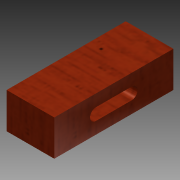
# Autodesk Inventor part: tensioner_wood_block(twb)
Saved by Autodesk Inventor 2015 SP1 (Build 190203100, 203)
## iProperties
Created: 2015-10-09
Part Number: tensioner_wood_block(twb)
Material: Wood (Oak)
Document SubType Name: Modeling
Designer: elilitwack
Density: 0.76 g/cm^3
Appearance: White Oak - Natural Medium Gloss
Mass: 20.4051 g
Surface Area: 77.8206 cm^2
Volume: 26.8488 cm^3
Author: elilitwack
Autodesk Inventor part; units mm, degrees
ref_plane "YZ Plane" through (0, 0, 0) normal (1, 0, 0) x (0, 1, 0)
ref_plane "XZ Plane" through (0, 0, 0) normal (0, 1, 0) x (-1, 0, 0)
ref_plane "XY Plane" through (0, 0, 0) normal (0, 0, 1) x (1, 0, 0)
sketch "tensioner_wood_block_base_sketch" plane through (0, 0, 0) normal (0, 1, 0) x (-1, 0, 0)
  line L0 (0, 0) -> (25.4, 0)
  line L1 (25.4, 0) -> (25.4, -63.5)
  line L2 (25.4, -63.5) -> (0, -63.5)
  line L3 (0, -63.5) -> (0, 0)
  dimension "d0" = 25.4
  dimension "d1" = 63.5
  constraints: 8 end point, 2 parallel, 1 horizontal, 1 perpendicular
  measures "d0" distance of L1.end L2.end
  measures "d1" distance of L0.end L1.end
extrude "base_extrusion" add sketch "tensioner_wood_block_base_sketch" along normal blind 19.05
sketch "tensioner_sketch" plane through (-25.4, 0, -63.5) normal (-1, 0, 0) x (0, 0, 1)
  line L0 (41.275, 9.525) -> (22.225, 9.525) construction
  line L1 (41.275, 12.7) -> (22.225, 12.7)
  line L2 (22.225, 6.35) -> (41.275, 6.35)
  arc A0 (41.275, 6.35) -> (41.275, 12.7) centre (41.275, 9.525) ccw
  arc A1 (22.225, 12.7) -> (22.225, 6.35) centre (22.225, 9.525) ccw
  line L3 (63.5, 0) -> (63.5, 19.05) projected
  line L4 (63.5, 0) -> (0, 0) projected
  line L5 (31.75, 0) -> (31.75, 9.525) construction
  line L6 (31.75, 9.525) -> (31.75, 19.05) construction
  line L7 (0, 19.05) -> (63.5, 19.05) projected
  dimension "d4" = 22.225
  dimension "d5" = 19.05
  dimension "d6" = 6.35
  constraints: 12 end point, 4 point on circle, 4 tangent, 3 midpoint, 2 centre point, 1 collinear, 1 horizontal, 1 parallel
  measures "d4" distance from line of L3 L0.start
  measures "d5" distance of L0.start L0.end
  measures "d6" distance between parallel lines of L1 L2
extrude "tensioner" cut sketch "tensioner_sketch" against normal up to next
equation "\"d0\" = twb_width"
equation "\"d1\" = twb_height"
equation "\"d2\" = twb_length"
equation "\"d4\" = twb_tensioner_from_edge"
equation "\"d5\" = bp_tensioner_height"
equation "\"d6\" = bp_tensioner_width"
equation "\"d7\" = twb_length"
equation "\"bp_thickness\" = 3.048"
equation "\"bp_height\" = gb_mh_seperation + st_outer_diameter"
equation "\"bp_width\" = 6 * st_rivet_distance"
equation "\"bp_axle_height\" = magic_axle_offset + gb_axle_from_edge + gb_to_bottom_of_side_assembly"
equation "\"magic_axle_offset\" = 3.175"
equation "\"bp_tensioner_width\" = 6.35"
equation "\"bp_tensioner_height\" = 19.05"
equation "\"bp_tensioner_from_bottom\" = 50.8"
equation "\"bp_tensioner_from_side\" = 25.4"
equation "\"bp_tensioner_wood_mount_from_tensioner_top\" = 12.7"
equation "\"bp_tensioner_wood_mount_diameter\" = 6.35"
equation "\"gb_mh_seperation\" = 111.1504"
equation "\"gb_mh_diameter\" = 6.35"
equation "\"gb_axle_from_edge\" = 38.1"
equation "\"gb_width\" = 127"
equation "\"gb_bearing_diameter\" = 28.575"
equation "\"gb_to_bottom_of_side_assembly\" = 4.7752"
equation "\"rv_hole_diameter\" = 3.57187"
equation "\"st_outer_diameter\" = 25.4"
equation "\"st_wall_thickness\" = 6.35"
equation "\"st_length\" = 939.8"
equation "\"st_gbmh_from_center\" = 0.5 * gb_mh_seperation"
equation "\"st_cutout_depth_right\" = 342.9"
equation "\"st_cutout_depth_left\" = 342.9"
equation "\"st_rivet_distance\" = 19.05"
equation "\"so_inner_diameter\" = 6.35"
equation "\"so_wall_thickness\" = 3.048"
equation "\"so_length\" = 25.4"
equation "\"twb_width\" = st_outer_diameter"
equation "\"twb_length\" = bp_tensioner_width + 2 * twb_margin_on_each_side"
equation "\"twb_height\" = 2 * bp_tensioner_wood_mount_diameter + bp_tensioner_height + 2 * bp_tensioner_wood_mount_from_tensioner_top + twb_margin_on_each_side"
equation "\"twb_margin_on_each_side\" = 6.35"
equation "\"twb_tensioner_from_edge\" = -0.5 * bp_tensioner_height + 0.5 * twb_height"
body "Solid1"
